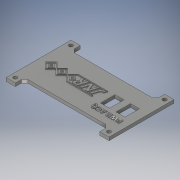
# Autodesk Inventor part: MapleMiniCase_TopCover
Saved by Autodesk Inventor 2018 (Build 220112000, 112)
## iProperties
Created: 2019-01-14
Part Number: MapleMiniCase_TopCover
Material: Generic
Document SubType Name: Modeling
Designer: tbrow
Density: 1 g/cm^3
Appearance: Default
Author: tbrow
## iProperties of the stored document MapleMiniCase_TopCover_3DPrint.ipt
Created: 2019-01-15
Part Number: MapleMiniCase_TopCover_3DPrint
Material: Generic
Document SubType Name: Modeling
Designer: tbrow
Density: 1 g/cm^3
Appearance: Default
Author: tbrow
Autodesk Inventor part; units mm, degrees
ref_plane "YZ Plane" through (0, 0, 0) normal (1, 0, 0) x (0, 1, 0)
ref_plane "XZ Plane" through (0, 0, 0) normal (0, 1, 0) x (-1, 0, 0)
ref_plane "XY Plane" through (0, 0, 0) normal (0, 0, 1) x (1, 0, 0)
sketch "Sketch1" plane through (0, 0, 0) normal (0, 1, 0) x (-1, 0, 0)
  line L0 (0, 0) -> (9.144, 0)
  line L1 (9.144, 0) -> (9.144, -9.144)
  line L2 (9.144, -9.144) -> (89.916, -9.144)
  line L3 (89.916, -9.144) -> (89.916, 0)
  line L4 (89.916, 0) -> (99.06, 0)
  line L5 (99.06, 0) -> (99.06, -58.6994)
  line L6 (99.06, -58.6994) -> (89.916, -58.6994)
  line L7 (89.916, -58.6994) -> (89.916, -49.5554)
  line L8 (89.916, -49.5554) -> (9.144, -49.5554)
  line L9 (9.144, -49.5554) -> (9.144, -58.6994)
  line L10 (9.144, -58.6994) -> (0, -58.6994)
  line L11 (0, -58.6994) -> (0, 0)
  dimension "d0" = 58.6994
  dimension "d1" = 9.144
  dimension "d2" = 9.144
  dimension "d3" = 9.144
  dimension "d4" = 9.144
  dimension "d5" = 9.144
  dimension "d7" = 9.144
  dimension "d16" = 99.06
  constraints: 24 end point, 8 perpendicular, 4 point on line, 2 horizontal
  measures "d0" distance of L4.end L5.end
  measures "d1" distance of L3.end L4.end
  measures "d2" distance of L2.end L3.end
  measures "d3" distance of L6.end L7.end
  measures "d4" distance of L0.start L0.end
  measures "d5" distance of L9.end L10.end
  measures "d7" distance of L5.end L6.end
  measures "d16" distance between parallel lines of L11 L5
extrude "Extrusion1" add sketch "Sketch1" along normal blind 3.175
sketch "Sketch2" plane through (0, 3.175, 0) normal (0, 1, 0) x (1, 0, 0)
  line L0 (-99.06, 0) -> (-89.916, 0) projected
  line L1 (-89.916, 58.6994) -> (-99.06, 58.6994) projected
  line L2 (-89.916, 49.5554) -> (-89.916, 58.6994) projected
  line L3 (-89.916, 0) -> (-89.916, 9.144) projected
  line L4 (-9.144, 0) -> (0, 0) projected
  line L5 (-9.144, 9.144) -> (-9.144, 0) projected
  line L6 (-9.144, 58.6994) -> (-9.144, 49.5554) projected
  circle A0 centre (-94.488, 4.572) radius 1.8542
  circle A1 centre (-94.488, 54.102) radius 1.8542
  circle A2 centre (-4.572, 54.102) radius 1.8542
  circle A3 centre (-4.572, 4.572) radius 1.8542
  line L7 (-99.06, 58.6994) -> (-99.06, 0) projected
  line L8 (0, 58.6994) -> (-9.144, 58.6994) projected
  line L9 (0, 0) -> (0, 58.6994) projected
  dimension "d10" = 3.7084
  dimension "d11" = 3.7084
  dimension "d12" = 3.7084
  dimension "d13" = 3.7084
  dimension "d17" = 4.572
  dimension "d18" = 4.5974
  dimension "d19" = 4.572
  dimension "d20" = 4.572
  dimension "d21" = 4.5974
  dimension "d22" = 4.572
  dimension "d23" = 4.572
  dimension "d24" = 4.572
  constraints: 4 centre point
  measures "d10" diameter of A0
  measures "d11" diameter of A1
  measures "d12" diameter of A2
  measures "d13" diameter of A3
  measures "d17" distance from line of L2 A1.centre
  measures "d18" distance from line of L1 A1.centre
  measures "d19" distance from line of L7 A0.centre
  measures "d20" distance from line of L0 A0.centre
  measures "d21" distance from line of L8 A2.centre
  measures "d22" distance from line of L9 A2.centre
  measures "d23" distance from line of L9 A3.centre
  measures "d24" distance from line of L4 A3.centre
extrude "Extrusion2" cut sketch "Sketch2" against normal blind 25.4
sketch "Sketch3" plane through (0, 3.175, 0) normal (0, 1, 0) x (1, 0, 0)
  line L0 (-33.274, 36.4617) -> (-24.384, 36.4617)
  line L1 (-24.384, 36.4617) -> (-24.384, 22.2377)
  line L2 (-24.384, 22.2377) -> (-33.274, 22.2377)
  line L3 (-33.274, 22.2377) -> (-33.274, 36.4617)
  line L4 (-18.034, 36.4617) -> (-9.144, 36.4617)
  line L5 (-9.144, 36.4617) -> (-9.144, 22.2377)
  line L6 (-9.144, 22.2377) -> (-18.034, 22.2377)
  line L7 (-18.034, 22.2377) -> (-18.034, 36.4617)
  line L8 (0, 0) -> (0, 58.6994) projected
  line L9 (0, 29.3497) -> (-99.06, 29.3497) construction
  line L10 (-99.06, 58.6994) -> (-99.06, 0) projected
  line L11 (-33.274, 29.3497) -> (-24.384, 29.3497) construction
  line L12 (-9.144, 29.3497) -> (-18.034, 29.3497) construction
  dimension "d25" = 14.224
  dimension "d26" = 8.89
  dimension "d27" = 8.89
  dimension "d28" = 6.35
  dimension "d32" = 9.144
  constraints: 22 end point, 6 midpoint, 4 parallel, 2 horizontal, 2 perpendicular, 2 point on line, 1 collinear
  measures "d25" distance of L2.end L0.start
  measures "d26" distance of L0.start L0.end
  measures "d27" distance of L4.start L4.end
  measures "d28" distance between parallel lines of L7 L1
  measures "d32" distance between parallel lines of L8 L5
extrude "Extrusion3" cut sketch "Sketch3" against normal blind 25.4
sketch "Sketch5" plane through (0, 3.175, 0) normal (0, 1, 0) x (1, 0, 0)
  line L0 (-7.0132, 13.6156) -> (-20.1648, 13.6156) construction
  line L1 (-20.1648, 13.6156) -> (-20.1648, 19.3396) construction
  line L2 (-20.1648, 19.3396) -> (-7.0132, 19.3396) construction
  line L3 (-7.0132, 19.3396) -> (-7.0132, 13.6156) construction
  line L4 (-24.384, 22.2377) -> (-33.274, 22.2377) projected
  line L5 (-13.589, 13.6156) -> (-13.589, 11.613) construction
  line L6 (-18.034, 22.2377) -> (-9.144, 22.2377) projected
  line L7 (-13.589, 22.2377) -> (-13.589, 19.0879) construction
  line L8 (-10.6511, 22.2377) -> (-10.6511, 9.144) construction
  line L9 (-89.916, 9.144) -> (-9.144, 9.144) projected
  line L10 (-10.6511, 15.6909) -> (6.071, 15.6909) construction
  line L11 (-24.3341, 13.528) -> (-33.3239, 13.528) construction
  line L12 (-33.3239, 13.528) -> (-33.3239, 20.194) construction
  line L13 (-33.3239, 20.194) -> (-24.3341, 20.194) construction
  line L14 (-24.3341, 20.194) -> (-24.3341, 13.528) construction
  line L15 (-33.274, 22.2377) -> (-33.274, 36.4617) projected
  line L16 (-28.829, 13.528) -> (-28.829, 6.1852) construction
  line L17 (-33.274, 22.2377) -> (-24.384, 22.2377) projected
  line L18 (-28.829, 22.2377) -> (-28.829, 19.0879) construction
  line L19 (-13.589, 17.4665) -> (-13.589, 15.0559) construction
  line L20 (-28.829, 17.4665) -> (-28.829, 17.4255) construction
  spline S0 degree 2 poles (-10.1004, 15.0168) (-10.1004, 15.3266) (-9.9022, 15.8885) (-9.7185, 16.0758) knots 0 0 0 1 2 2 2
  spline S1 degree 2 poles (-9.7185, 16.0758) (-9.6069, 16.1947) (-9.3331, 16.3892) (-9.171, 16.4576) knots 0 0 0 1 2 2 2
  spline S2 degree 2 poles (-9.171, 16.4576) (-9.0053, 16.5261) (-8.6199, 16.6053) (-8.3822, 16.6053) knots 0 0 0 1 2 2 2
  line L21 (-8.3822, 16.6053) -> (-7.7986, 16.6053)
  line L22 (-7.7986, 16.6053) -> (-7.7986, 18.0606)
  line L23 (-7.7986, 18.0606) -> (-6.682, 18.0606)
  line L24 (-6.682, 18.0606) -> (-6.682, 13.6156)
  line L25 (-6.682, 13.6156) -> (-8.4074, 13.6156)
  spline S3 degree 2 poles (-8.4074, 13.6156) (-8.7892, 13.6156) (-9.3475, 13.7561) (-9.5745, 13.9074) knots 0 0 0 1 2 2 2
  spline S4 degree 2 poles (-9.5745, 13.9074) (-9.8266, 14.0767) (-10.1004, 14.6314) (-10.1004, 15.0168) knots 0 0 0 1 2 2 2
  spline S5 degree 2 poles (-8.9549, 15.0456) (-8.9549, 14.8547) (-8.7748, 14.5846) (-8.6523, 14.5341) knots 0 0 0 1 2 2 2
  spline S6 degree 2 poles (-8.6523, 14.5341) (-8.4938, 14.4657) (-8.2057, 14.4441) (-7.9571, 14.4441) knots 0 0 0 1 2 2 2
  line L26 (-7.9571, 14.4441) -> (-7.7986, 14.4441)
  line L27 (-7.7986, 14.4441) -> (-7.7986, 15.7768)
  line L28 (-7.7986, 15.7768) -> (-7.8779, 15.7768)
  spline S7 degree 2 poles (-7.8779, 15.7768) (-8.0327, 15.7768) (-8.3137, 15.7696) (-8.4182, 15.7516) knots 0 0 0 1 2 2 2
  spline S8 degree 2 poles (-8.4182, 15.7516) (-8.5082, 15.7372) (-8.7063, 15.6508) (-8.7604, 15.5967) knots 0 0 0 1 2 2 2
  spline S9 degree 2 poles (-8.7604, 15.5967) (-8.8756, 15.4887) (-8.9549, 15.2473) (-8.9549, 15.0456) knots 0 0 0 1 2 2 2
  line L29 (-16.4293, 13.6156) -> (-15.3054, 18.0606)
  line L30 (-15.3054, 18.0606) -> (-14.0807, 18.0606)
  line L31 (-14.0807, 18.0606) -> (-13.3675, 15.3122)
  line L32 (-13.3675, 15.3122) -> (-12.6795, 18.0606)
  line L33 (-12.6795, 18.0606) -> (-11.4511, 18.0606)
  line L34 (-11.4511, 18.0606) -> (-10.3273, 13.6156)
  line L35 (-10.3273, 13.6156) -> (-11.4872, 13.6156)
  line L36 (-11.4872, 13.6156) -> (-12.0995, 16.5909)
  line L37 (-12.0995, 16.5909) -> (-12.8416, 13.6156)
  line L38 (-12.8416, 13.6156) -> (-13.951, 13.6156)
  line L39 (-13.951, 13.6156) -> (-14.657, 16.5945)
  line L40 (-14.657, 16.5945) -> (-15.2982, 13.6156)
  line L41 (-15.2982, 13.6156) -> (-16.4293, 13.6156)
  line L42 (-21.0868, 18.0606) -> (-19.7288, 18.0606)
  line L43 (-19.7288, 18.0606) -> (-18.4933, 16.4288)
  line L44 (-18.4933, 16.4288) -> (-18.0898, 16.4288)
  line L45 (-18.0898, 16.4288) -> (-18.0898, 18.0606)
  line L46 (-18.0898, 18.0606) -> (-16.9804, 18.0606)
  line L47 (-16.9804, 18.0606) -> (-16.9804, 13.6156)
  line L48 (-16.9804, 13.6156) -> (-18.767, 13.6156)
  spline S10 degree 2 poles (-18.767, 13.6156) (-19.138, 13.6156) (-19.6856, 13.7092) (-19.9197, 13.8533) knots 0 0 0 1 2 2 2
  spline S11 degree 2 poles (-19.9197, 13.8533) (-20.1574, 14.0046) (-20.4384, 14.4765) (-20.4384, 14.8367) knots 0 0 0 1 2 2 2
  spline S12 degree 2 poles (-20.4384, 14.8367) (-20.4384, 15.3446) (-19.9773, 15.9822) (-19.5919, 16.1695) knots 0 0 0 1 2 2 2
  line L49 (-19.5919, 16.1695) -> (-21.0868, 18.0606)
  spline S13 degree 2 poles (-19.2929, 14.9772) (-19.2929, 14.8079) (-19.1633, 14.5665) (-19.0156, 14.5017) knots 0 0 0 1 2 2 2
  spline S14 degree 2 poles (-19.0156, 14.5017) (-18.9111, 14.4585) (-18.6554, 14.4333) (-18.4645, 14.4333) knots 0 0 0 1 2 2 2
  line L50 (-18.4645, 14.4333) -> (-18.0898, 14.4333)
  line L51 (-18.0898, 14.4333) -> (-18.0898, 15.6292)
  line L52 (-18.0898, 15.6292) -> (-18.4104, 15.6292)
  spline S15 degree 2 poles (-18.4104, 15.6292) (-18.641, 15.6292) (-18.9687, 15.5715) (-19.0804, 15.4815) knots 0 0 0 1 2 2 2
  spline S16 degree 2 poles (-19.0804, 15.4815) (-19.1885, 15.395) (-19.2929, 15.1645) (-19.2929, 14.9772) knots 0 0 0 1 2 2 2
  line L53 (-22.3236, 18.0667) -> (-23.8257, 13.6217)
  line L54 (-23.8257, 13.6217) -> (-25.0432, 13.6217)
  line L55 (-25.0432, 13.6217) -> (-26.5453, 18.0667)
  line L56 (-26.5453, 18.0667) -> (-25.3962, 18.0667)
  line L57 (-25.3962, 18.0667) -> (-25.1188, 17.1589)
  line L58 (-25.1188, 17.1589) -> (-23.7212, 17.1589)
  line L59 (-23.7212, 17.1589) -> (-23.4402, 18.0667)
  line L60 (-23.4402, 18.0667) -> (-22.3236, 18.0667)
  line L61 (-24.8739, 16.3521) -> (-24.42, 14.8824)
  line L62 (-24.42, 14.8824) -> (-23.9626, 16.3521)
  line L63 (-23.9626, 16.3521) -> (-24.8739, 16.3521)
  spline S17 degree 2 poles (-28.9046, 18.1531) (-27.9033, 18.1531) (-26.729, 16.9428) (-26.729, 15.8478) knots 0 0 0 1 2 2 2
  spline S18 degree 2 poles (-26.729, 15.8478) (-26.729, 14.7924) (-27.9069, 13.5352) (-28.9082, 13.5352) knots 0 0 0 1 2 2 2
  spline S19 degree 2 poles (-28.9082, 13.5352) (-29.1712, 13.5352) (-29.5962, 13.5965) (-29.7908, 13.6469) knots 0 0 0 1 2 2 2
  spline S20 degree 2 poles (-29.7908, 13.6469) (-29.9421, 13.6937) (-30.2987, 13.8486) (-30.4103, 13.9062) knots 0 0 0 1 2 2 2
  line L64 (-30.4103, 13.9062) -> (-30.4103, 14.9653)
  line L65 (-30.4103, 14.9653) -> (-30.2987, 14.9653)
  spline S21 degree 2 poles (-30.2987, 14.9653) (-30.2158, 14.8932) (-29.9709, 14.6915) (-29.816, 14.5978) knots 0 0 0 1 2 2 2
  spline S22 degree 2 poles (-29.816, 14.5978) (-29.6611, 14.5006) (-29.2901, 14.3673) (-29.0847, 14.3673) knots 0 0 0 1 2 2 2
  spline S23 degree 2 poles (-29.0847, 14.3673) (-28.8434, 14.3673) (-28.4436, 14.5186) (-28.2599, 14.7095) knots 0 0 0 1 2 2 2
  spline S24 degree 2 poles (-28.2599, 14.7095) (-28.0942, 14.8788) (-27.8816, 15.4587) (-27.8816, 15.8514) knots 0 0 0 1 2 2 2
  spline S25 degree 2 poles (-27.8816, 15.8514) (-27.8816, 16.2656) (-28.1014, 16.8311) (-28.2815, 17.004) knots 0 0 0 1 2 2 2
  spline S26 degree 2 poles (-28.2815, 17.004) (-28.4544, 17.1733) (-28.8794, 17.321) (-29.092, 17.321) knots 0 0 0 1 2 2 2
  spline S27 degree 2 poles (-29.092, 17.321) (-29.3117, 17.321) (-29.7115, 17.1733) (-29.8484, 17.0833) knots 0 0 0 1 2 2 2
  spline S28 degree 2 poles (-29.8484, 17.0833) (-29.9997, 16.9932) (-30.2266, 16.8023) (-30.3095, 16.7267) knots 0 0 0 1 2 2 2
  line L66 (-30.3095, 16.7267) -> (-30.4103, 16.7267)
  line L67 (-30.4103, 16.7267) -> (-30.4103, 17.7713)
  spline S29 degree 2 poles (-30.4103, 17.7713) (-30.2879, 17.8289) (-29.9673, 17.973) (-29.7944, 18.0234) knots 0 0 0 1 2 2 2
  spline S30 degree 2 poles (-29.7944, 18.0234) (-29.5854, 18.0883) (-29.2216, 18.1531) (-28.9046, 18.1531) knots 0 0 0 1 2 2 2
  spline S31 degree 2 poles (-35.1075, 19.241) (-34.9274, 19.2842) (-34.5672, 19.3274) (-34.1817, 19.3274) knots 0 0 0 1 2 2 2
  spline S32 degree 2 poles (-34.1817, 19.3274) (-33.8323, 19.3274) (-33.3388, 19.1509) (-33.1731, 18.9888) knots 0 0 0 1 2 2 2
  spline S33 degree 2 poles (-33.1731, 18.9888) (-33.011, 18.8303) (-32.8453, 18.3981) (-32.8345, 18.1459) knots 0 0 0 1 2 2 2
  spline S34 degree 2 poles (-32.8345, 18.1459) (-31.8944, 18.1027) (-30.8102, 16.8816) (-30.8102, 15.8442) knots 0 0 0 1 2 2 2
  spline S35 degree 2 poles (-30.8102, 15.8442) (-30.8102, 14.7743) (-31.9556, 13.528) (-32.9606, 13.528) knots 0 0 0 1 2 2 2
  spline S36 degree 2 poles (-32.9606, 13.528) (-33.962, 13.528) (-35.1147, 14.7671) (-35.1147, 15.8442) knots 0 0 0 1 2 2 2
  spline S37 degree 2 poles (-35.1147, 15.8442) (-35.1147, 16.6294) (-34.4627, 17.7533) (-33.8647, 17.991) knots 0 0 0 1 2 2 2
  spline S38 degree 2 poles (-33.8647, 17.991) (-33.8719, 18.3188) (-34.1493, 18.5674) (-34.4951, 18.5674) knots 0 0 0 1 2 2 2
  spline S39 degree 2 poles (-34.4951, 18.5674) (-34.632, 18.5674) (-34.931, 18.4881) (-34.9958, 18.4521) knots 0 0 0 1 2 2 2
  line L68 (-34.9958, 18.4521) -> (-35.1075, 18.4521)
  line L69 (-35.1075, 18.4521) -> (-35.1075, 19.241)
  spline S40 degree 2 poles (-33.663, 16.968) (-33.8071, 16.7735) (-33.962, 16.2584) (-33.962, 15.8406) knots 0 0 0 1 2 2 2
  spline S41 degree 2 poles (-33.962, 15.8406) (-33.962, 15.4443) (-33.7999, 14.886) (-33.6594, 14.7059) knots 0 0 0 1 2 2 2
  spline S42 degree 2 poles (-33.6594, 14.7059) (-33.5189, 14.5258) (-33.1587, 14.3673) (-32.9642, 14.3673) knots 0 0 0 1 2 2 2
  spline S43 degree 2 poles (-32.9642, 14.3673) (-32.7589, 14.3673) (-32.4239, 14.515) (-32.269, 14.7023) knots 0 0 0 1 2 2 2
  spline S44 degree 2 poles (-32.269, 14.7023) (-32.1321, 14.8752) (-31.9628, 15.4479) (-31.9628, 15.8442) knots 0 0 0 1 2 2 2
  spline S45 degree 2 poles (-31.9628, 15.8442) (-31.9628, 16.2512) (-32.1249, 16.7915) (-32.2654, 16.9752) knots 0 0 0 1 2 2 2
  spline S46 degree 2 poles (-32.2654, 16.9752) (-32.4059, 17.1589) (-32.7697, 17.3174) (-32.9642, 17.3174) knots 0 0 0 1 2 2 2
  spline S47 degree 2 poles (-32.9642, 17.3174) (-33.1623, 17.3174) (-33.5297, 17.1481) (-33.663, 16.968) knots 0 0 0 1 2 2 2
  point P0 (0, 0)
  dimension "d34" = 270
  dimension "d35" = 270
  constraints: 16 end point, 7 vertical, 5 midpoint, 4 collinear, 2 point on line, 1 horizontal, 4 other
emboss "Emboss1" sketch "Sketch5" operation add depth 0.508 direction (0, -1, 0)
sketch "Sketch6" plane through (0, 3.175, 0) normal (0, 1, 0) x (1, 0, 0)
  line L0 (-40.3703, 23.4244) -> (-65.0308, 23.4244)
  line L1 (-67.6978, 24.2626) -> (-40.3703, 24.2626)
  line L2 (-40.3703, 24.2626) -> (-40.3703, 23.4244)
  line L3 (-56.7722, 24.8976) -> (-54.7334, 24.8976) construction
  line L4 (-37.8303, 42.2014) -> (-37.8303, 16.4839) construction
  line L5 (-37.2178, 34.4226) -> (-67.6978, 34.4226)
  line L6 (-67.6978, 34.4226) -> (-67.6978, 35.2481) construction
  line L7 (-67.6978, 35.2481) -> (-37.2178, 35.2481)
  line L8 (-37.2178, 35.2481) -> (-37.2178, 34.4226)
  line L9 (-51.6068, 33.7876) -> (-53.7536, 33.7876) construction
  line L10 (-64.8178, 29.3426) -> (-67.9608, 26.1995)
  line L11 (-67.9608, 26.1995) -> (-71.1039, 29.3426)
  line L12 (-71.1039, 29.3426) -> (-67.9608, 32.4857)
  line L13 (-67.9608, 32.4857) -> (-64.8178, 29.3426)
  line L14 (-67.9608, 26.1995) -> (-67.9608, 32.4857) construction
  line L15 (-69.4875, 29.3426) -> (-67.9608, 27.816)
  line L16 (-67.9608, 27.816) -> (-66.4342, 29.3426)
  line L17 (-66.4342, 29.3426) -> (-67.9608, 30.8693)
  line L18 (-67.9608, 30.8693) -> (-69.4875, 29.3426)
  line L19 (-65.0308, 23.4244) -> (-67.9608, 23.4244)
  line L20 (-67.6978, 35.2481) -> (-67.9609, 35.2481)
  line L21 (-73.2268, 28.6904) -> (-73.2268, 24.4371) construction
  line L22 (-81.6359, 29.3426) -> (-78.4928, 26.1995)
  line L23 (-78.4928, 27.816) -> (-80.0195, 29.3426)
  line L24 (-76.9662, 29.3426) -> (-78.4928, 27.816)
  line L25 (-78.4928, 26.1995) -> (-75.3497, 29.3426)
  line L26 (-75.3497, 29.3426) -> (-78.4928, 32.4857)
  line L27 (-78.4928, 30.8693) -> (-76.9662, 29.3426)
  line L28 (-80.0195, 29.3426) -> (-78.4928, 30.8693)
  line L29 (-78.4928, 32.4857) -> (-81.6359, 29.3426)
  line L30 (-83.7588, 28.6904) -> (-83.7588, 23.2318) construction
  line L31 (-85.8817, 29.3426) -> (-89.0248, 26.1995)
  line L32 (-89.0248, 26.1995) -> (-92.1679, 29.3426)
  line L33 (-90.5514, 29.3426) -> (-89.0248, 27.816)
  line L34 (-89.0248, 27.816) -> (-87.4982, 29.3426)
  line L35 (-92.1679, 29.3426) -> (-89.0248, 32.4857)
  line L36 (-89.0248, 30.8693) -> (-90.5514, 29.3426)
  line L37 (-87.4982, 29.3426) -> (-89.0248, 30.8693)
  line L38 (-89.0248, 32.4857) -> (-85.8817, 29.3426)
  line L39 (-88.9961, 24.5544) -> (-93.7843, 29.3426)
  line L40 (-89.0355, 23.4137) -> (-94.9581, 29.3363)
  line L41 (-88.9961, 34.1309) -> (-93.7843, 29.3426)
  line L42 (-89.0355, 35.2589) -> (-94.9581, 29.3363)
  line L43 (-78.4928, 35.2481) -> (-83.7588, 29.9821)
  line L44 (-84.2078, 29.3426) -> (-88.9961, 24.5544)
  line L45 (-78.4928, 34.1596) -> (-83.3098, 29.3426)
  line L46 (-83.7588, 28.6904) -> (-89.0355, 23.4137)
  line L47 (-78.4928, 24.5257) -> (-83.3098, 29.3426)
  line L48 (-83.7588, 29.9821) -> (-89.0355, 35.2589)
  line L49 (-78.4928, 23.4244) -> (-83.7588, 28.6904)
  line L50 (-84.2078, 29.3426) -> (-88.9961, 34.1309)
  line L51 (-67.9608, 23.4244) -> (-73.2268, 28.6904)
  line L52 (-73.6759, 29.3426) -> (-78.4928, 34.1596)
  line L53 (-67.6978, 24.2626) -> (-72.7778, 29.3426)
  line L54 (-73.2268, 29.9821) -> (-78.4928, 35.2481)
  line L55 (-67.6978, 34.4226) -> (-72.7778, 29.3426)
  line L56 (-73.2268, 28.6904) -> (-78.4928, 23.4244)
  line L57 (-67.9609, 35.2481) -> (-73.2268, 29.9821)
  line L58 (-73.6759, 29.3426) -> (-78.4928, 24.5257)
  line L59 (-89.916, 58.6994) -> (-99.06, 58.6994) projected
  line L60 (-33.274, 22.2377) -> (-33.274, 36.4617) projected
  line L61 (-44.2866, 24.2626) -> (-44.2866, 34.4226) construction
  line L62 (-44.2866, 29.3426) -> (-40.1094, 29.3426) construction
  line L63 (-33.274, 29.3497) -> (-111.4558, 29.3497) construction
  line L64 (-39.2583, 25.0026) -> (-65.7075, 25.0026) construction
  line L65 (-65.7075, 25.0026) -> (-65.7075, 34.711) construction
  line L66 (-65.7075, 34.711) -> (-39.2583, 34.711) construction
  line L67 (-39.2583, 34.711) -> (-39.2583, 25.0026) construction
  line L68 (-89.916, 9.144) -> (-9.144, 9.144) projected
  line L69 (-53.5411, 25.0026) -> (-53.5411, 24.2626) construction
  spline S0 degree 2 poles (-45.1794, 30.363) (-44.5774, 32.1525) (-42.2766, 34.0493) (-40.7097, 34.0493) knots 0 0 0 1 2 2 2
  spline S1 degree 2 poles (-40.7097, 34.0493) (-40.0087, 34.0493) (-39.4892, 33.8019) knots 0 0 0 1 1 1
  line L70 (-39.4892, 33.8019) -> (-40.1324, 31.9299)
  spline S2 degree 2 poles (-40.1324, 31.9299) (-40.5118, 32.3175) (-41.155, 32.3175) knots 0 0 0 1 1 1
  spline S3 degree 2 poles (-41.155, 32.3175) (-42.524, 32.3175) (-43.2167, 30.2805) knots 0 0 0 1 1 1
  line L71 (-43.2167, 30.2805) -> (-45.0062, 25.0026)
  line L72 (-45.0062, 25.0026) -> (-47.002, 25.0026)
  line L73 (-47.002, 25.0026) -> (-45.1794, 30.363)
  line L74 (-53.9292, 33.8926) -> (-51.9088, 33.8926)
  line L75 (-51.9088, 33.8926) -> (-50.144, 28.3013)
  spline S4 degree 2 poles (-50.144, 28.3013) (-49.9873, 27.8147) (-49.9461, 27.5673) knots 0 0 0 1 1 1
  line L76 (-49.9461, 27.5673) -> (-49.9213, 27.5673)
  spline S5 degree 2 poles (-49.9213, 27.5673) (-49.8141, 28.0374) (-49.4842, 29.0023) knots 0 0 0 1 1 1
  line L77 (-49.4842, 29.0023) -> (-47.8266, 33.8926)
  line L78 (-47.8266, 33.8926) -> (-45.9299, 33.8926)
  line L79 (-45.9299, 33.8926) -> (-48.9564, 25.0026)
  line L80 (-48.9564, 25.0026) -> (-51.1088, 25.0026)
  line L81 (-51.1088, 25.0026) -> (-52.7994, 30.4125)
  spline S6 degree 2 poles (-52.7994, 30.4125) (-52.9149, 30.7836) (-52.9974, 31.1382) knots 0 0 0 1 1 1
  line L82 (-52.9974, 31.1382) -> (-53.0221, 31.1382)
  spline S7 degree 2 poles (-53.0221, 31.1382) (-53.0798, 30.833) (-53.3932, 29.9177) knots 0 0 0 1 1 1
  line L83 (-53.3932, 29.9177) -> (-55.059, 25.0026)
  line L84 (-55.059, 25.0026) -> (-56.9558, 25.0026)
  line L85 (-56.9558, 25.0026) -> (-53.9292, 33.8926)
  line L86 (-63.4295, 33.8926) -> (-61.1287, 33.8926)
  line L87 (-61.1287, 33.8926) -> (-60.5266, 31.6082)
  spline S8 degree 2 poles (-60.5266, 31.6082) (-60.4607, 31.3443) (-60.3122, 30.932) (-60.1143, 30.6434) (-59.8504, 30.4867) (-59.669, 30.4867) knots 0 0 0 1 2 3 4 4 4
  line L88 (-59.669, 30.4867) -> (-59.1329, 30.4867)
  line L89 (-59.1329, 30.4867) -> (-57.9701, 33.8926)
  line L90 (-57.9701, 33.8926) -> (-55.9662, 33.8926)
  line L91 (-55.9662, 33.8926) -> (-58.9927, 25.0026)
  line L92 (-58.9927, 25.0026) -> (-62.1677, 25.0026)
  spline S9 degree 2 poles (-62.1677, 25.0026) (-65.4005, 25.0026) (-64.584, 27.4189) knots 0 0 0 1 1 1
  spline S10 degree 2 poles (-64.584, 27.4189) (-64.4191, 27.8807) (-63.8666, 28.6724) (-63.1326, 29.3074) (-62.242, 29.761) (-61.7472, 29.8929) knots 0 0 0 1 2 3 4 4 4
  line L93 (-61.7472, 29.8929) -> (-61.7389, 29.9177)
  spline S11 degree 2 poles (-61.7389, 29.9177) (-61.9121, 29.9836) (-62.1925, 30.2558) (-62.4069, 30.6269) (-62.5801, 31.0557) (-62.6461, 31.2619) knots 0 0 0 1 2 3 4 4 4
  line L94 (-62.6461, 31.2619) -> (-63.4295, 33.8926)
  line L95 (-60.4854, 26.5035) -> (-59.6442, 28.9775)
  line L96 (-59.6442, 28.9775) -> (-60.5101, 28.9775)
  spline S12 degree 2 poles (-60.5101, 28.9775) (-61.1534, 28.9775) (-61.6729, 28.6064) knots 0 0 0 1 1 1
  spline S13 degree 2 poles (-61.6729, 28.6064) (-62.2007, 28.2271) (-62.3904, 27.6663) knots 0 0 0 1 1 1
  spline S14 degree 2 poles (-62.3904, 27.6663) (-62.7862, 26.5035) (-61.3925, 26.5035) knots 0 0 0 1 1 1
  line L97 (-61.3925, 26.5035) -> (-60.4854, 26.5035)
  point P0 (0, 0)
  dimension "d39" = 0.8382
  dimension "d40" = 0.635
  dimension "d41" = 2.54
  dimension "d42" = 30.48
  dimension "d43" = 0.635
  dimension "d44" = 0.8255
  dimension "d45" = 45
  dimension "d46" = 10.16
  dimension "d47" = 5.08
  dimension "d48" = 4.445
  dimension "d49" = 4.445
  dimension "d50" = 26.9875
  dimension "d51" = 1.143
  dimension "d52" = 0.8345
  dimension "d53" = 1.143
  dimension "d54" = 0.8255
  dimension "d55" = 1.143
  dimension "d56" = 0
  dimension "d59" = 270
  constraints: 126 end point, 35 parallel, 16 symmetric about line, 5 perpendicular, 4 point on line, 2 horizontal, 2 midpoint, 5 other
  measures "d39" distance of L1.end L0.start
  measures "d40" distance between parallel lines of L1 L3
  measures "d41" distance between parallel lines of L4 L2
  measures "d42" distance of L20.start L7.end
  measures "d43" distance between parallel lines of L5 L9
  measures "d44" distance of L55.start L20.start
  measures "d45" angle of L5 L13
  measures "d46" distance between parallel lines of L5 L1
  measures "d47" distance from line of L1 L13.end
  measures "d48" distance of L13.end L14.start
  measures "d49" distance of L12.end L13.end
  measures "d50" distance from line of L4 L13.end
  measures "d51" distance between parallel lines of L11 L15
  measures "d52" distance between parallel lines of L40 L39
  measures "d53" distance between parallel lines of L39 L32
  measures "d54" distance between parallel lines of L42 L41
  measures "d55" distance between parallel lines of L35 L41
  measures "d56" horizontal distance of L19.end L14.start
emboss "Emboss2" sketch "Sketch6" operation add depth 0.762 direction (0, -1, 0)
sketch "Sketch7" plane through (0, 3.175, 0) normal (0, 1, 0) x (1, 0, 0)
  line L0 (-40.1324, 31.9299) -> (-39.4892, 33.8019) projected
  line L1 (-40.1324, 31.9299) -> (-44.2029, 20.0837)
  line L2 (-39.4892, 33.8019) -> (-37.418, 39.8295)
  line L3 (-37.418, 39.8295) -> (-35.9996, 37.5718)
  line L4 (-35.9996, 37.5718) -> (-36.7079, 19.7852)
  line L5 (-36.7079, 19.7852) -> (-44.2029, 20.0837)
  point P0 (0, 0)
  constraints: 10 end point, 2 collinear, 1 perpendicular
extrude "Extrusion4" cut sketch "Sketch7" along normal blind 25.4
chamfer "Chamfer1" distance 3.175 angle 45 4 edges at (-89.916, 1.5875, -49.5554) (-9.144, 1.5875, -49.5554) (-9.144, 1.5875, -9.144) (-89.916, 1.5875, -9.144)
move faces "Move1" translate (0, 0, 2.667) faces at (-37.1263, 1.0583, -9.144) (-89.916, 1.0583, -3.9793) (-94.5627, 1.0583, -6.4247) (-92.964, 1.0583, 0) (-2.7238, 1.0583, -4.4228) (-3.048, 1.0583, 0) (-11.2607, 1.0583, -8.0857) (-9.144, 1.0583, -1.9897) (-88.8577, 1.0583, -7.0273)
move faces "Move2" translate (0, 0, -2.667) faces at (-61.9337, 1.0583, -49.5554) (-92.6398, 1.0583, -53.9528) (-96.012, 1.0583, -58.6994) (-11.2607, 1.0583, -50.6137) (-9.144, 1.0583, -54.7201) (-6.096, 1.0583, -58.6994) (-2.7238, 1.0583, -53.9528) (-88.8577, 1.0583, -51.6721) (-89.916, 1.0583, -56.7097)
move faces "Move3" translate (-2.54, 0, 0) faces at (-93.0057, 2.1167, -55.6551) (-96.012, 1.0583, -61.3664) (-88.8577, 1.0583, -54.3391) (-89.916, 2.1167, -57.3871) (-94.4133, 1.0583, -3.7577) (-89.916, 2.1167, -1.3123) (-96.012, 2.1167, 2.667) (-88.8577, 1.0583, -4.3603) (-99.06, 1.0583, -18.6775)
equation "\"d2\" = d1"
equation "\"d3\" = d1"
equation "\"d4\" = d1"
equation "\"d5\" = d1"
equation "\"d7\" = d1"
equation "\"d19\" = d17"
equation "\"d20\" = d17"
equation "\"d22\" = d17"
equation "\"d23\" = d17"
equation "\"d24\" = d17"
body "Solid1"
